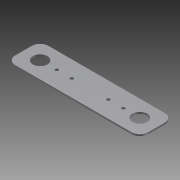
# Autodesk Inventor part: sketch femur 6 cm
Saved by Autodesk Inventor 2012 (Build 160160000, 160)
## iProperties
Created: 2012-12-04
Part Number: sketch femur 6 cm
Material: Default
Document SubType Name: Modeling
Designer: irwan
Density: 1 g/cm^3
Author: irwan
Autodesk Inventor part; units mm, degrees
ref_plane "YZ Plane" through (0, 0, 0) normal (1, 0, 0) x (0, 1, 0)
ref_plane "XZ Plane" through (0, 0, 0) normal (0, 1, 0) x (-1, 0, 0)
ref_plane "XY Plane" through (0, 0, 0) normal (0, 0, 1) x (1, 0, 0)
sketch "Sketch1" plane through (0, 0, 0) normal (0, 0, 1) x (1, 0, 0)
  circle A0 centre (-124.2929, 102.2868) radius 4.385
  circle A1 centre (-64.2929, 102.2868) radius 4.385
  line L0 (-116.2929, 112.2868) -> (-59.2929, 112.2868)
  line L1 (-129.2929, 92.2868) -> (-59.2929, 92.2868)
  line L2 (-124.3591, 92.2868) -> (-129.2929, 92.2868)
  line L3 (-134.2929, 107.2868) -> (-134.2929, 97.2868)
  line L4 (-54.2929, 97.2868) -> (-54.2929, 107.2868)
  arc A2 (-129.2929, 112.2868) -> (-134.2929, 107.2868) centre (-129.2929, 107.2868) ccw
  arc A3 (-134.2929, 97.2868) -> (-129.2929, 92.2868) centre (-129.2929, 97.2868) ccw
  arc A4 (-59.2929, 92.2868) -> (-54.2929, 97.2868) centre (-59.2929, 97.2868) ccw
  arc A5 (-54.2929, 107.2868) -> (-59.2929, 112.2868) centre (-59.2929, 107.2868) ccw
  line L5 (-59.2929, 112.2868) -> (-72.2929, 112.2868)
  line L6 (-116.2929, 112.2868) -> (-129.2929, 112.2868)
  circle A6 centre (-114.2929, 102.2868) radius 1
  circle A7 centre (-105.2929, 102.2868) radius 1
  circle A8 centre (-74.2929, 102.2868) radius 1
  circle A9 centre (-83.2929, 102.2868) radius 1
  point P0 (-126.1429, 102.2868)
  point P1 (-79.2929, 92.2868)
  dimension "d109" = 10
  dimension "d110" = 10
  dimension "d111" = 8.77
  dimension "d112" = 8.77
  dimension "d113" = 2
  dimension "d114" = 2
  dimension "d115" = 10
  dimension "d116" = 9
  dimension "d117" = 2
  dimension "d118" = 2
  dimension "d119" = 10
  dimension "d120" = 9
  dimension "d121" = 60
  dimension "d126" = 10
  dimension "d401" = 20
  constraints: 14 end point, 10 centre point, 9 tangent, 8 point on circle, 3 collinear, 3 equal radius, 2 parallel, 2 point on line, 1 perpendicular
  measures "d109" distance from line of L3 A0.centre
  measures "d110" distance from line of L4 A1.centre
  measures "d111" diameter of A0
  measures "d112" diameter of A1
  measures "d113" diameter of A6
  measures "d114" diameter of A7
  measures "d115" distance of A6.centre A0.centre
  measures "d116" distance of A7.centre A6.centre
  measures "d117" diameter of A8
  measures "d118" diameter of A9
  measures "d119" distance of A8.centre A1.centre
  measures "d120" distance of A9.centre A8.centre
  measures "d121" distance of A1.centre A0.centre
  measures "d126" distance from line of L1 A1.centre
  measures "d401" distance between parallel lines of L1 L0
extrude "Extrusion1" add sketch "Sketch1" along normal blind 1
body "Solid1"
